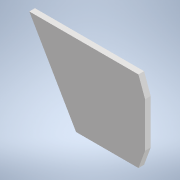
# Autodesk Inventor part: Деталь4
Saved by Autodesk Inventor 2021.2 (Build 252289000, 289)
## iProperties
Created: 2021-10-12
Part Number: Деталь4
Material: Типовые
Document SubType Name: Modeling
Designer: Surflay
Density: 1 g/cm^3
Appearance: По умолчанию
Author: Surflay
Autodesk Inventor part; units mm, degrees
ref_plane "YZ Plane" through (0, 0, 0) normal (1, 0, 0) x (0, 1, 0)
ref_plane "XZ Plane" through (0, 0, 0) normal (0, 1, 0) x (-1, 0, 0)
ref_plane "XY Plane" through (0, 0, 0) normal (0, 0, 1) x (1, 0, 0)
sketch "Эскиз1" plane through (0, 0, 0) normal (0, 0, 1) x (1, 0, 0)
  line L0 (0, 0) -> (247, 0)
  line L1 (247, 0) -> (247, 6.4)
  line L2 (0, 6.4) -> (247, 6.4)
  line L3 (0, 0) -> (0, 6.4)
  line L4 (85.1893, 28.9) -> (77, 6.4)
  line L5 (85.1893, 83.9) -> (85.1893, 28.9)
  line L6 (77, 106.4) -> (85.1893, 83.9)
  line L7 (238.8107, 106.4) -> (77, 106.4)
  line L8 (0, 6.4) -> (-61.5, 112.9211)
  line L9 (-61.5, 112.9211) -> (-166.5, 112.9211)
  line L10 (77, 6.4) -> (0, 6.4)
  line L11 (-57.735, 106.4) -> (77, 106.4)
  line L12 (85.1893, 83.9) -> (85.1893, 28.9)
  line L13 (77, 106.4) -> (85.1893, 83.9)
  line L14 (85.1893, 28.9) -> (77, 6.4)
  line L15 (0, 6.4) -> (-57.735, 106.4)
extrude "Выдавливание1" add sketch "Эскиз1" along normal blind 7 contours L8 L11 L6 L5 L4 L2
